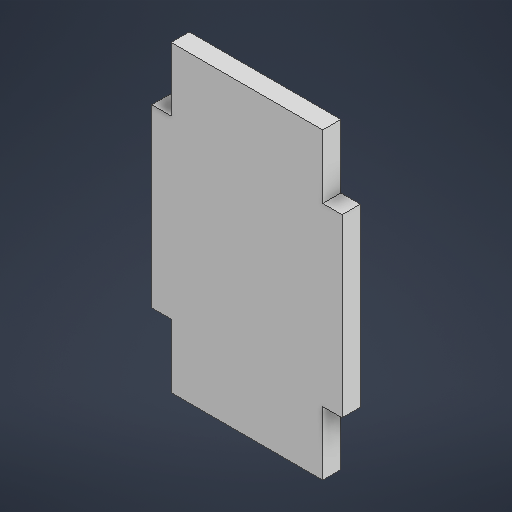
# Autodesk Inventor part: Backboard
Saved by Autodesk Inventor 2027 (Build 310192000, 192)
## iProperties
Created: 2026-05-09
Part Number: Backboard
Material: Generic
Document SubType Name: Modeling
Designer: alexy
Density: 1 g/cm^3
Appearance: Default
Author: alexy
Autodesk Inventor part; units mm, degrees
ref_plane "YZ Plane" through (0, 0, 0) normal (1, 0, 0) x (0, 1, 0)
ref_plane "XZ Plane" through (0, 0, 0) normal (0, 1, 0) x (-1, 0, 0)
ref_plane "XY Plane" through (0, 0, 0) normal (0, 0, 1) x (1, 0, 0)
sketch "Sketch1" plane through (0, 0, 0) normal (0, 0, 1) x (1, 0, 0)
  line L0 (0, 0) -> (25, 0)
  line L1 (25, 0) -> (25, 50)
  line L2 (25, 50) -> (0, 50)
  line L3 (0, 50) -> (0, 0)
  line L4 (-3.2, 39.5) -> (0, 39.5)
  line L5 (0, 39.5) -> (0, 10.5)
  line L6 (0, 10.5) -> (-3.2, 10.5)
  line L7 (-3.2, 10.5) -> (-3.2, 39.5)
  line L8 (-3.2, 39.5) -> (0, 10.5) construction
  line L9 (0, 39.5) -> (-3.2, 10.5) construction
  line L10 (28.2, 39.5) -> (25, 39.5)
  line L11 (25, 39.5) -> (25, 10.5)
  line L12 (25, 10.5) -> (28.2, 10.5)
  line L13 (28.2, 10.5) -> (28.2, 39.5)
  line L14 (28.2, 39.5) -> (25, 10.5) construction
  line L15 (25, 39.5) -> (28.2, 10.5) construction
  point P0 (-1.6, 25)
  point P1 (26.6, 25)
  point P2 (0, 25)
  point P3 (0, 39.5)
  dimension "d0" = 25
  dimension "d1" = 50
  dimension "d2" = 3.2
  dimension "d3" = 3.2
  dimension "d4" = 29
  dimension "d5" = 29
  constraints: 32 end point, 6 parallel, 5 midpoint, 3 horizontal, 3 perpendicular, 2 horizontal alignment, 2 point on line
  measures "d0" distance of L2.end L1.end
  measures "d1" distance of L0.end L1.end
  measures "d2" distance of L11.end L12.end
  measures "d3" distance of L5.end L6.end
  measures "d4" distance of L6.end L4.start
  measures "d5" distance of L12.end L10.start
extrude "Extrusion1" add sketch "Sketch1" along normal blind 3
body "Solid1"
